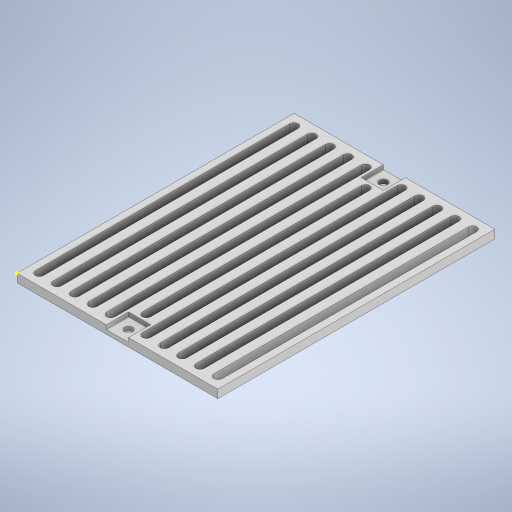
# Autodesk Inventor part: Tray middle
Saved by Autodesk Inventor 2024 (Build 280153000, 153)
## iProperties
Created: 2023-11-19
Part Number: Tray middle
Material: Generic
Document SubType Name: Modeling
Designer: olson
Density: 1 g/cm^3
Appearance: Default
Author: olson
Autodesk Inventor part; units mm, degrees
ref_plane "YZ Plane" through (0, 0, 0) normal (1, 0, 0) x (0, 1, 0)
ref_plane "XZ Plane" through (0, 0, 0) normal (0, 1, 0) x (-1, 0, 0)
ref_plane "XY Plane" through (0, 0, 0) normal (0, 0, 1) x (1, 0, 0)
sketch "Sketch1" plane through (0, 0, 0) normal (0, 1, 0) x (-1, 0, 0)
  line L0 (0, 0) -> (-72.5, 0)
  line L1 (-72.5, 0) -> (-72.5, -100)
  line L2 (-72.5, -100) -> (0, -100)
  line L3 (0, -100) -> (0, 0)
  dimension "d0" = 72.5
  dimension "d1" = 100
  constraints: 8 end point, 2 parallel, 1 horizontal, 1 perpendicular
  measures "d0" distance of L2.end L1.end
  measures "d1" distance of L1.end L0.end
extrude "Extrusion1" add sketch "Sketch1" along normal blind 3
sketch "Sketch11" plane through (0, 3, 0) normal (0, 1, 0) x (1, 0, 0)
  point P0 (0, 0)
sketch "Sketch13" plane through (0, 3, 0) normal (0, 1, 0) x (1, 0, 0)
  line L0 (0, 0) -> (72.5, 0) projected
  line L1 (36.25, 0) -> (36.25, 8)
  line L2 (36.25, 8) -> (32.25, 8)
  line L3 (32.25, 8) -> (32.25, 0)
  line L4 (36.25, 0) -> (32.25, 0)
  line L5 (36.25, 0) -> (40.25, 0)
  line L6 (40.25, 0) -> (40.25, 8)
  line L7 (40.25, 8) -> (36.25, 8)
  line L8 (72.5, 100) -> (0, 100) projected
  line L9 (36.25, 100) -> (32.25, 100)
  line L10 (32.25, 100) -> (32.25, 92)
  line L11 (32.25, 92) -> (40.25, 92)
  line L12 (40.25, 92) -> (40.25, 100)
  line L13 (40.25, 100) -> (36.25, 100)
  line L14 (72.5, 0) -> (72.5, 100) projected
  dimension "d190" = 8
  dimension "d191" = 4
  dimension "d192" = 4
  dimension "d193" = 8
  constraints: 24 end point, 9 point on line, 5 perpendicular, 2 midpoint, 1 collinear, 1 horizontal, 1 vertical
  measures "d190" distance of L1.start L1.end
  measures "d191" distance of L1.end L2.end
  measures "d192" distance of L1.start L5.end
  measures "d193" distance of L9.end L10.end
extrude "Extrusion11" cut sketch "Sketch13" against normal blind 1.5
sketch "Sketch14" plane through (0, 1.5, 0) normal (0, 1, 0) x (1, 0, 0)
  line L0 (0, 0) -> (72.5, 0) projected
  line L1 (40.25, 8) -> (32.25, 8)
  line L2 (32.25, 8) -> (32.25, 0)
  line L3 (32.25, 0) -> (40.25, 0)
  line L4 (40.25, 0) -> (40.25, 8)
  line L5 (72.5, 100) -> (0, 100) projected
  line L6 (40.25, 100) -> (32.25, 100)
  line L7 (32.25, 100) -> (32.25, 92)
  line L8 (32.25, 92) -> (40.25, 92)
  line L9 (40.25, 92) -> (40.25, 100)
  line L10 (72.5, 46) -> (64.5, 46) projected
  line L11 (64.5, 46) -> (64.5, 54) projected
  line L12 (72.5, 46) -> (64.5, 46)
  line L13 (64.5, 46) -> (64.5, 54)
  line L14 (64.5, 54) -> (72.5, 54)
  line L15 (72.5, 54) -> (72.5, 46)
  circle A0 centre (36.25, 4) radius 1.5
  circle A1 centre (36.25, 96) radius 1.5
  circle A2 centre (68.5, 50) radius 1.5
  dimension "d199" = 8
  dimension "d200" = 8
  dimension "d201" = 3
  dimension "d202" = 3
  dimension "d203" = 3
  constraints: 24 end point, 6 parallel, 4 point on line, 3 centre point, 3 horizontal, 3 perpendicular
  measures "d199" distance of L3.end L2.end
  measures "d200" distance of L7.end L6.end
  measures "d201" diameter of A0
  measures "d202" diameter of A1
  measures "d203" diameter of A2
extrude "Extrusion12" cut sketch "Sketch14" against normal blind 1.5 contours A0 | A1 | A2
sketch "Sketch15" plane through (0, 3, 0) normal (0, 1, 0) x (1, 0, 0)
  circle A0 centre (36.25, 4) radius 1.5 projected
  line L0 (0, 100) -> (0, 0) projected
  circle A1 centre (36.25, 96) radius 1.5 projected
  line L1 (32.25, 8) -> (40.25, 8) projected
  arc A2 (2.5, 4) -> (5.5, 4) centre (4, 4) ccw
  arc A3 (15.4, 4) -> (18.4, 4) centre (16.9, 4) ccw
  arc A4 (21.85, 4) -> (24.85, 4) centre (23.35, 4) ccw
  arc A5 (28.3, 4) -> (31.3, 4) centre (29.8, 4) ccw
  arc A6 (41.2, 4) -> (44.2, 4) centre (42.7, 4) ccw
  arc A7 (47.65, 4) -> (50.65, 4) centre (49.15, 4) ccw
  arc A8 (54.1, 4) -> (57.1, 4) centre (55.6, 4) ccw
  arc A9 (60.55, 4) -> (63.55, 4) centre (62.05, 4) ccw
  arc A10 (67, 4) -> (70, 4) centre (68.5, 4) ccw
  arc A11 (70, 96) -> (67, 96) centre (68.5, 96) ccw
  arc A12 (63.55, 96) -> (60.55, 96) centre (62.05, 96) ccw
  arc A13 (57.1, 96) -> (54.1, 96) centre (55.6, 96) ccw
  arc A14 (50.65, 96) -> (47.65, 96) centre (49.15, 96) ccw
  arc A15 (44.2, 96) -> (41.2, 96) centre (42.7, 96) ccw
  arc A16 (31.3, 96) -> (28.3, 96) centre (29.8, 96) ccw
  arc A17 (24.85, 96) -> (21.85, 96) centre (23.35, 96) ccw
  arc A18 (18.4, 96) -> (15.4, 96) centre (16.9, 96) ccw
  arc A19 (5.5, 96) -> (2.5, 96) centre (4, 96) ccw
  line L2 (8.95, 16.45) -> (8.95, 83.55)
  line L3 (11.95, 83.55) -> (11.95, 16.45)
  line L4 (15.4, 4) -> (15.4, 96)
  line L5 (18.4, 96) -> (18.4, 4)
  line L6 (21.85, 96) -> (21.85, 4)
  line L7 (24.85, 4) -> (24.85, 96)
  line L8 (28.3, 96) -> (28.3, 4)
  line L9 (31.3, 4) -> (31.3, 96)
  line L10 (41.2, 96) -> (41.2, 4)
  line L11 (44.2, 4) -> (44.2, 96)
  line L12 (47.65, 96) -> (47.65, 4)
  line L13 (50.65, 4) -> (50.65, 96)
  line L14 (54.1, 96) -> (54.1, 4)
  line L15 (57.1, 4) -> (57.1, 96)
  line L16 (60.55, 96) -> (60.55, 4)
  line L17 (63.55, 4) -> (63.55, 96)
  line L18 (67, 43.55) -> (67, 4)
  line L19 (70, 4) -> (70, 43.55)
  line L20 (67, 56.45) -> (67, 96)
  line L21 (70, 96) -> (70, 56.45)
  line L22 (36.25, 4) -> (36.25, 10.45)
  arc A20 (34.75, 10.45) -> (37.75, 10.45) centre (36.25, 10.45) ccw
  line L23 (36.25, 96) -> (36.25, 89.55)
  arc A21 (37.75, 89.55) -> (34.75, 89.55) centre (36.25, 89.55) ccw
  line L24 (34.75, 10.45) -> (34.75, 89.55)
  line L25 (37.75, 89.55) -> (37.75, 10.45)
  arc A22 (8.95, 4) -> (11.95, 4) centre (10.45, 4) ccw
  arc A23 (11.95, 96) -> (8.95, 96) centre (10.45, 96) ccw
  line L26 (8.95, 96) -> (8.95, 83.55)
  line L27 (11.95, 96) -> (11.95, 83.55)
  line L28 (8.95, 16.45) -> (8.95, 4)
  line L29 (11.95, 16.45) -> (11.95, 4)
  line L30 (5.5, 4) -> (5.5, 43.55)
  line L31 (5.5, 56.45) -> (5.5, 96)
  line L32 (2.5, 96) -> (2.5, 56.45)
  line L33 (2.5, 43.55) -> (2.5, 4)
  line L34 (2.5, 56.45) -> (2.5, 43.55)
  line L35 (5.5, 43.55) -> (5.5, 56.45)
  line L36 (67, 56.45) -> (67, 43.55)
  line L37 (70, 43.55) -> (70, 56.45)
  dimension "d216" = 3
  dimension "d217" = 3
  dimension "d218" = 3
  dimension "d219" = 3
  dimension "d220" = 3
  dimension "d221" = 3
  dimension "d225" = 3
  dimension "d226" = 3
  dimension "d227" = 3
  dimension "d228" = 3
  dimension "d229" = 3
  dimension "d230" = 3
  dimension "d231" = 3
  dimension "d232" = 3
  dimension "d233" = 3
  dimension "d242" = 6.45
  dimension "d243" = 3
  dimension "d244" = 6.45
  dimension "d245" = 3
  dimension "d248" = 3
  dimension "d249" = 3
  constraints: 72 end point, 44 point on circle, 22 centre point, 21 tangent, 5 parallel, 5 point on line, 4 vertical, 2 coincident, 2 collinear
  measures "d216" diameter of A2
  measures "d217" diameter of A3
  measures "d218" diameter of A4
  measures "d219" diameter of A5
  measures "d220" diameter of A6
  measures "d221" diameter of A7
  measures "d225" diameter of A11
  measures "d226" diameter of A12
  measures "d227" diameter of A13
  measures "d228" diameter of A14
  measures "d229" diameter of A15
  measures "d230" diameter of A16
  measures "d231" diameter of A17
  measures "d232" diameter of A18
  measures "d233" diameter of A19
  measures "d242" distance of L22.start L22.end
  measures "d243" diameter of A20
  measures "d244" distance of L23.start L23.end
  measures "d245" diameter of A21
  measures "d248" diameter of A22
  measures "d249" diameter of A23
extrude "Extrusion13" cut sketch "Sketch15" against normal blind 3 contours A20 L24 A21 L25 | L33 L34 L32 A19 L31 L35 L30 A2 | L4 A18 L5 A3 | L6 A17 L7 A4 | L8 A16 L9 A5 | L10 A15 L11 A6 | L12 A14 L13 A7 | L14 A13 L15 A8 | L16 A12 L17 A9 | L18 L36 L20 A11 L21 L37 L19 A10 | L2 L26 A23 L27 L3 L29 A22 L28
sketch "Sketch16" plane through (0, 3, 0) normal (0, 1, 0) x (1, 0, 0)
  point P0 (0, 0)
body "Solid1"
